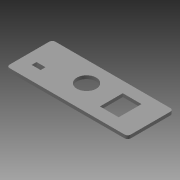
# Autodesk Inventor part: rearPlate_jack
Saved by Autodesk Inventor 2016 (Build 200138000, 138)
## iProperties
Created: 2017-03-04
Part Number: rearPlate_jack
Material: Generic
Document SubType Name: Modeling
Designer: Tyler
Density: 1 g/cm^3
Appearance: Default
Author: Tyler
Autodesk Inventor part; units mm, degrees
ref_plane "YZ Plane" through (0, 0, 0) normal (1, 0, 0) x (0, 1, 0)
ref_plane "XZ Plane" through (0, 0, 0) normal (0, 1, 0) x (-1, 0, 0)
ref_plane "XY Plane" through (0, 0, 0) normal (0, 0, 1) x (1, 0, 0)
sketch "Sketch1" plane through (0, 0, 0) normal (0, 0, 1) x (1, 0, 0)
  line L0 (-29.75, -11.25) -> (29.75, -11.25)
  line L1 (29.75, -11.25) -> (29.75, 11.25)
  line L2 (29.75, 11.25) -> (-29.75, 11.25)
  line L3 (-29.75, 11.25) -> (-29.75, -11.25)
  line L4 (-29.75, -11.25) -> (29.75, 11.25) construction
  line L5 (29.75, -11.25) -> (-29.75, 11.25) construction
  point P0 (0, 0)
  dimension "d0" = 59.5
  dimension "d1" = 22.5
  constraints: 12 end point, 2 midpoint, 2 parallel, 1 horizontal, 1 perpendicular
  measures "d0" distance of L2.end L1.end
  measures "d1" distance of L0.end L1.end
extrude "Extrusion1" add sketch "Sketch1" against normal blind 1.6
fillet "Fillet1" radius 1.5 4 edges at (29.75, 11.25, -0.8) (29.75, -11.25, -0.8) (-29.75, 11.25, -0.8) (-29.75, -11.25, -0.8)
sketch "Sketch2" plane through (0, 0, 0) normal (0, 0, 1) x (1, 0, 0)
  circle A0 centre (-2.949, 1.26) radius 4.75
  line L0 (-28.25, -11.25) -> (28.25, -11.25) projected
  line L1 (-29.75, 9.75) -> (-29.75, -9.75) projected
  line L2 (-24.199, -4.44) -> (-19.799, -4.44)
  line L3 (-19.799, -4.44) -> (-19.799, -2.04)
  line L4 (-19.799, -2.04) -> (-24.199, -2.04)
  line L5 (-24.199, -2.04) -> (-24.199, -4.44)
  line L6 (-24.199, -4.44) -> (-19.799, -2.04) construction
  line L7 (-19.799, -4.44) -> (-24.199, -2.04) construction
  point P0 (0, 0)
  point P1 (-28.349, -5.24)
  point P2 (-21.999, -3.24)
  dimension "d5" = 9.5
  dimension "d15" = 12.51
  dimension "d16" = 26.801
  dimension "d17" = 6.01
  dimension "d18" = 1.401
  dimension "d19" = 4.4
  dimension "d20" = 2.4
  dimension "d21" = 6.35
  dimension "d22" = 2
  constraints: 12 end point, 2 midpoint, 2 parallel, 1 centre point, 1 horizontal, 1 perpendicular
  measures "d5" diameter of A0
  measures "d15" distance from line of L0 A0.centre
  measures "d16" distance from line of A0.centre L1
  measures "d17" distance from line of L0 point (-28.349, -5.24)
  measures "d18" distance from line of L1 point (-28.349, -5.24)
  measures "d19" distance of L4.end L3.end
  measures "d20" distance of L3.end L2.end
  measures "d21" horizontal distance of point (-21.999, -3.24) point (-28.349, -5.24)
  measures "d22" vertical distance of point (-28.349, -5.24) point (-21.999, -3.24)
extrude "Extrusion2" cut sketch "Sketch2" against normal through all
sketch "Sketch4" plane through (0, 0, 0) normal (0, 0, 1) x (1, 0, 0)
  line L0 (-28.25, -11.25) -> (28.25, -11.25) projected
  line L1 (-29.75, 9.75) -> (-29.75, -9.75) projected
  line L2 (10.231, -5.34) -> (19.431, -5.34)
  line L3 (19.431, -5.34) -> (19.431, 5.86)
  line L4 (19.431, 5.86) -> (10.231, 5.86)
  line L5 (10.231, 5.86) -> (10.231, -5.34)
  line L6 (10.231, -5.34) -> (19.431, 5.86) construction
  line L7 (19.431, -5.34) -> (10.231, 5.86) construction
  point P0 (0, 0)
  point P1 (-28.349, -5.24)
  point P2 (14.831, 0.26)
  dimension "d23" = 6.01
  dimension "d24" = 1.401
  dimension "d25" = 9.2
  dimension "d26" = 11.2
  dimension "d28" = 43.18
  dimension "d29" = 0.1
  constraints: 12 end point, 2 midpoint, 2 parallel, 1 horizontal, 1 perpendicular
  measures "d23" distance from line of L0 point (-28.349, -5.24)
  measures "d24" distance from line of L1 point (-28.349, -5.24)
  measures "d25" distance of L4.end L3.end
  measures "d26" distance of L3.end L2.end
  measures "d28" horizontal distance of point (14.831, 0.26) point (-28.349, -5.24)
  measures "d29" distance from line of L2 point (-28.349, -5.24)
extrude "Extrusion4" cut sketch "Sketch4" against normal through all
body "Solid1"
